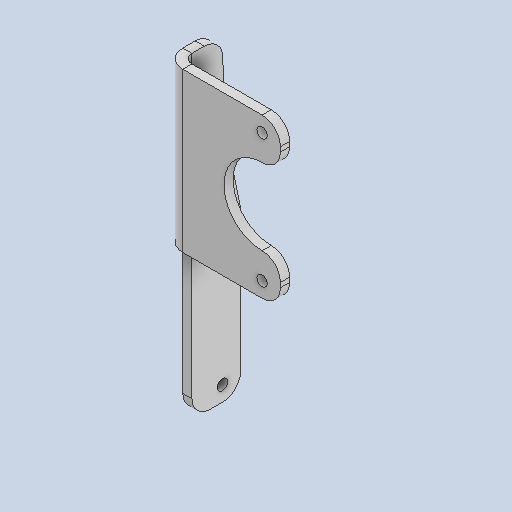
# Autodesk Inventor part: hipjoint_toleg_under_right
Saved by Autodesk Inventor 2024.1 (Build 281209000, 209)
## iProperties
Created: 2024-10-09
Part Number: hipjoint_toleg_under_right
Material: 一般
Document SubType Name: Sheet Metal
Designer: hibik
Density: 1 g/cm^3
Sheet Metal Rule: Default_mm
Appearance: 既定
Author: hibik
Autodesk Inventor part; units mm, degrees
ref_plane "YZ Plane" through (0, 0, 0) normal (1, 0, 0) x (0, 1, 0)
ref_plane "XZ Plane" through (0, 0, 0) normal (0, 1, 0) x (-1, 0, 0)
ref_plane "XY Plane" through (0, 0, 0) normal (0, 0, 1) x (1, 0, 0)
sketch "スケッチ1" plane through (0, 0, 0) normal (0, 0, 1) x (1, 0, 0)
  circle A0 centre (0, 0) radius 6.25
  line L0 (0, 13) -> (-16, 13)
  line L1 (-16, 13) -> (-16, -13)
  line L2 (-16, -13) -> (0, -13)
  line L3 (0, -13) -> (0, 13)
  line L4 (0, 13) -> (3, 13)
  line L5 (3, 13) -> (3, -13)
  line L6 (3, -13) -> (0, -13)
  line L7 (0, -13) -> (0, 13)
  point P0 (-16, 0)
  point P1 (3, -5.4829)
  point P2 (3, 5.4829)
  dimension "d0" = 12.5
  dimension "d1" = 16
  dimension "d2" = 26
  dimension "d3" = 3
  measures "d0" diameter of A0
  measures "d1" distance of L2.end L1.end
  measures "d2" distance of L1.end L0.end
  measures "d3" distance of L5.end L6.end
extrude "プレート1" add sketch "スケッチ1" along normal blind 1.5 contours A0 L3 L4 L5 | L5 L6 L3 A0 | A0 L3 L2 L1 L0
sketch "スケッチ2" plane through (-14.5, 13, 1.5) normal (-1, 0, 0) x (0, -1, 0)
  line L0 (26, 0) -> (0, 0)
  line L1 (0, 0) -> (0, -11)
  line L2 (0, -11) -> (26, -11)
  line L3 (26, -11) -> (26, 0)
  constraints: 6 end point, 1 horizontal, 1 perpendicular, 1 vertical
edge flange "フランジ1" height 11 angle 90 thickness 1.5 bend radius 1.5 thickness toward (-1, 0, 0) relief straight relief width 1.5 relief depth 0.75 edges at (-16, 0, 0) wall of the first edge with corners at (-14.5, -13, 1.5) (-14.5, 13, 1.5) (-14.5, 13, -9.5) (-14.5, -13, -9.5)
bend "曲げ1"
corner "コーナー1"
sketch "スケッチ3" plane through (-16, -13, -9.5) normal (-1, 0, 0) x (0, 0, 1)
  line L0 (8, 0) -> (0, 0) projected
  line L1 (0, 0) -> (8, 0)
  line L2 (8, 0) -> (8, -26)
  line L3 (8, -26) -> (0, -26)
  line L4 (0, -26) -> (0, 0)
  line L5 (8, 0) -> (8, 26) projected
  arc A0 (0, 0) -> (3, 26) centre (-111.1667, 26) ccw
  line L6 (3, 20) -> (3, 26) construction
  line L7 (0, 26) -> (8, 26) projected
  line L8 (0, 0) -> (0, 26) projected
  point P0 (9.5, 13)
  point P1 (8, 0)
  dimension "d15" = 26
  dimension "d21" = 5
  constraints: 10 end point, 2 parallel, 2 point on circle, 1 centre point, 1 collinear, 1 horizontal, 1 perpendicular, 1 point on line, 1 tangent, 1 vertical
  measures "d15" distance of L3.end L0.end
  measures "d21" distance between parallel lines of L5 L6
sheet face with bend "面2" sketch "スケッチ3" thickness 1.5 toward (1, 0, 0) bend radius 1.5 relief straight relief width 1.5 relief depth 0.75 contours L2 L3 L4 L0
bend "曲げ2"
extrude "切り取り1" cut sketch "スケッチ3" against normal blind 1.5 contours L8 L7 A0
sketch "スケッチ5" plane through (0, 0, 0) normal (0, 0, -1) x (-1, 0, 0)
  circle A0 centre (0, 10.5) radius 0.85 projected
  circle A1 centre (0, -10.5) radius 0.85 projected
  point P0 (0, 0)
extrude "切り取り2" cut sketch "スケッチ5" against normal blind 1.5
sketch "スケッチ6" plane through (-16, -39, -1.5) normal (-1, 0, 0) x (0, 0, 1)
  circle A0 centre (-5, 23.5) radius 0.85 projected
  circle A1 centre (-5, 2.5) radius 0.85 projected
  point P0 (1.5, 39)
extrude "切り取り3" cut sketch "スケッチ6" against normal blind 1.5
fillet "フィレット1" radius 3 8 edges at (3, 13, 0.75) (3, 5.4829, 0.75) (3, -5.4829, 0.75) (3, -13, 0.75) (-15.25, -13, -9.5) (-15.25, 13, -6.5) (-15.25, -39, -9.5) (-15.25, -39, -1.5)
equation "\"d23\" = Thickness"
equation "\"d25\" = Thickness"
equation "\"d27\" = Thickness"
equation "\"d4\" = Thickness"
equation "\"d5\" = BendReliefWidth"
equation "\"d6\" = BendReliefDepth"
equation "\"d7\" = MinimumRemnant"
equation "\"d8\" = TransitionRadius"
equation "\"d11\" = BendRadius"
equation "\"d12\" = CornerReliefSize"
equation "\"d13\" = GapSize"
equation "\"d14\" = JacobiRadiusSize"
equation "\"d16\" = BendRadius"
equation "\"d17\" = BendReliefWidth"
equation "\"d19\" = MinimumRemnant"
equation "\"d18\" = BendReliefDepth"
equation "\"d20\" = TransitionRadius"
equation "\"BendRadius\" = Thickness"
equation "\"BendReliefWidth\" = Thickness"
equation "\"BendReliefDepth\" = 0.5 * Thickness"
equation "\"CornerReliefSize\" = 4 * Thickness"
equation "\"MinimumRemnant\" = 2 * Thickness"
equation "\"TransitionRadius\" = BendRadius"
equation "\"JacobiRadiusSize\" = BendRadius"
equation "\"GapSize\" = Thickness"
equation "\"Thickness\" = 1.5"
